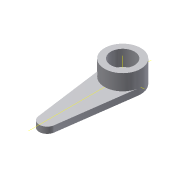
# Autodesk Inventor part: empty
Saved by Autodesk Inventor 2014 (Build 180170000, 170)
## iProperties
Created: 2015-04-13
Part Number: empty
Material: Generic
Document SubType Name: Modeling
Designer: Martin
Density: 1 g/cm^3
Appearance: Default
Author: Martin
Autodesk Inventor part; units mm, degrees
ref_plane "YZ Plane" through (0, 0, 0) normal (1, 0, 0) x (0, 1, 0)
ref_plane "XZ Plane" through (0, 0, 0) normal (0, 1, 0) x (-1, 0, 0)
ref_plane "XY Plane" through (0, 0, 0) normal (0, 0, 1) x (1, 0, 0)
sketch "Sketch1" plane through (0, 0, 0) normal (0, 0, 1) x (1, 0, 0)
  circle A0 centre (0, 0) radius 1.875
  circle A1 centre (0, 0) radius 2.875
  line L0 (-2.8489, -0.3866) -> (0, -21.3815) construction
  line L1 (0, -21.3815) -> (2.8489, -0.3866) construction
  line L2 (0, -26.2328) -> (0, 7.7263) projected
  line L3 (-4.025, 0) -> (4.025, 0) projected
  arc A2 (-1.25, -12.1696) -> (1.25, -12.1696) centre (0, -12) ccw
  line L4 (-1.25, -12.1696) -> (-2.8489, -0.3866)
  line L5 (1.25, -12.1696) -> (2.8489, -0.3866)
  dimension "d0" = 3.75
  dimension "d1" = 1
  dimension "d2" = 12
  dimension "d3" = 2.5
  constraints: 8 end point, 7 tangent, 5 point on circle, 3 centre point, 3 point on line, 2 coincident, 2 collinear
  measures "d0" diameter of A0
  measures "d1" radial gap between concentric circles of A1 A0
  measures "d2" distance of A2.centre point (0, 0)
  measures "d3" distance of L5.start L4.start
extrude "Extrusion1" add sketch "Sketch1" against normal blind 1
extrude "Extrusion2" add sketch "Sketch1" along normal blind 2.5 contours L3 A1 L2 A0 | A0 L2 A1 L3 | A0 L3 A1 L2 | L2 A1 L3 A0
body "Solid1"
